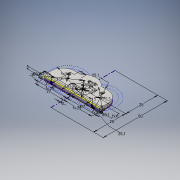
# Autodesk Inventor part: mount2
Saved by Autodesk Inventor 2016 (Build 200138000, 138)
## iProperties
Created: 2016-12-01
Part Number: mount2
Material: 一般
Document SubType Name: Modeling
Designer: KOTA-NPC2
Density: 1 g/cm^3
Appearance: 既定
Author: KOTA-NPC2
Autodesk Inventor part; units mm, degrees
ref_plane "YZ Plane" through (0, 0, 0) normal (1, 0, 0) x (0, 1, 0)
ref_plane "XZ Plane" through (0, 0, 0) normal (0, 1, 0) x (-1, 0, 0)
ref_plane "XY Plane" through (0, 0, 0) normal (0, 0, 1) x (1, 0, 0)
sketch "構築線" plane through (0, 0, 0) normal (0, 0, 1) x (1, 0, 0)
  circle A0 centre (0, 0) radius 8.5
  circle A1 centre (0, 0) radius 2.8 construction
  circle A2 centre (0, 0) radius 5 construction
  line L0 (0, -8.6) -> (-25, -8.6) construction
  line L1 (0, -11.6) -> (-25, -11.6) construction
  circle A3 centre (-12.8148, 0.95) radius 10.05 construction
  circle A4 centre (-12.8148, 0.95) radius 12.55 construction
  circle A5 centre (0, 5) radius 0.8
  circle A6 centre (-4.3301, 2.5) radius 0.8
  circle A7 centre (-4.3301, -2.5) radius 0.8
  circle A8 centre (0, -5) radius 0.8
  circle A9 centre (4.3301, -2.5) radius 0.8
  circle A10 centre (4.3301, 2.5) radius 0.8
  line L2 (25, -8.6) -> (0, -8.6) construction
  circle A11 centre (12.8148, 0.95) radius 10.05 construction
  circle A12 centre (12.8148, 0.95) radius 12.55 construction
  line L3 (0, -11.6) -> (25, -11.6) construction
  line L4 (-22, -8.6) -> (-22, -2.6)
  arc A13 (-13, 6.4) -> (-22, -2.6) centre (-13, -2.6) ccw
  line L5 (-13, 6.4) -> (-8, 6.4)
  line L6 (-22, -8.6) -> (0, -8.6)
  line L7 (0, 25) -> (0, -25)
  line L8 (0, -8.6) -> (22, -8.6)
  line L9 (22, -8.6) -> (22, -2.6)
  arc A14 (8, 6.4) -> (-8, 6.4) centre (0, 0) ccw
  line L10 (8, 6.4) -> (13, 6.4)
  arc A15 (22, -2.6) -> (13, 6.4) centre (13, -2.6) ccw
  circle A16 centre (0, 0) radius 3
  circle A17 centre (0, 0) radius 1
  circle A18 centre (12.8148, 0.95) radius 1.05
  circle A19 centre (-12.8148, 0.95) radius 1.05
  circle A20 centre (12.8148, 0.95) radius 2.75
  circle A21 centre (-12.8148, 0.95) radius 2.75
  dimension "d0" = 17
  dimension "d1" = 5.6
  dimension "d2" = 10
  dimension "d12" = 25
  dimension "d13" = 8.6
  dimension "d14" = 0
  dimension "d17" = 0
  dimension "d18" = 25
  dimension "d19" = 3
  dimension "d22" = 20.1
  dimension "d23" = 25.1
  dimension "d29" = 1.6
  dimension "d30" = 0
  dimension "d31" = 5
  dimension "d34" = 360
  dimension "d38" = 25
  dimension "d41" = 20.1
  dimension "d42" = 25.1
  dimension "d43" = 25
  dimension "d46" = 22
  dimension "d47" = 6
  dimension "d48" = 5
  dimension "d49" = 50
  dimension "d50" = 25
  dimension "d51" = 25
  dimension "d52" = 22
  dimension "d53" = 6
  dimension "d56" = 15
  dimension "d57" = 15
  dimension "d58" = 6
  dimension "d59" = 2
  dimension "d99" = 2.1
  dimension "d100" = 2.1
  dimension "d105" = 5.5
  dimension "d106" = 5.5
  constraints: 22 centre point, 22 end point, 10 coincident, 8 tangent, 7 horizontal, 6 point on circle, 2 concentric, 2 vertical, 1 collinear, 1 perpendicular, 1 point on line, 13 other
  measures "d0" diameter of A0
  measures "d1" diameter of A1
  measures "d2" diameter of A2
  measures "d12" distance of L0.start L0.end
  measures "d13" distance from line of point (0, 0) L0
  measures "d14" horizontal distance of point (0, 0) L0.start
  measures "d17" horizontal distance of L1.start point (0, 0)
  measures "d18" distance of L1.start L1.end
  measures "d19" distance between parallel lines of L1 L0
  measures "d22" diameter of A3
  measures "d23" diameter of A4
  measures "d29" diameter of A5
  measures "d30" horizontal distance of point (0, 0) A5.centre
  measures "d31" distance of point (0, 0) A5.centre
  measures "d38" distance of L0.start L2.start
  measures "d41" diameter of A11
  measures "d42" diameter of A12
  measures "d43" distance of L1.start L3.end
  measures "d46" distance of L0.start L4.start
  measures "d47" distance of L4.start L4.end
  measures "d48" distance of L5.start L5.end
  measures "d49" distance of L7.start L7.end
  measures "d50" distance of point (0, 0) L7.start
  measures "d51" distance of L7.end point (0, 0)
  measures "d52" distance of L0.start L8.end
  measures "d53" distance of L8.end L9.end
  measures "d56" distance between parallel lines of L8 L10
  measures "d57" distance between parallel lines of L6 L5
  measures "d58" diameter of A16
  measures "d59" diameter of A17
  measures "d99" diameter of A18
  measures "d100" diameter of A19
  measures "d105" diameter of A20
  measures "d106" diameter of A21
extrude "外形作成" add sketch "構築線" along normal blind 2.5 and the other way blind 1 contours A0 L7 A8 A16 A5 | A0 L7 A14 L10 A15 L9 L8 | L7 A5 A16 A8 A0 | A0 L7 L6 L4 A13 L5 A14 | A16 L7 A17 | L7 A17 A16 | A18 | A19 | A20 | A21
extrude "押し出し4" cut sketch "構築線" against normal blind 1 contours A0 L7 A8 A16 A5 | L7 A5 A16 A8 A0 | A16 L7 A17 | L7 A17 A16
sketch "固定具" plane through (-22, -8.6, 2.5) normal (0, -1, 0) x (1, 0, 0)
  circle A0 centre (6, -2) radius 1.05
  line L0 (0, 0) -> (0, -3.5) projected
  line L1 (0, 0) -> (44, 0) projected
  circle A1 centre (38, -2) radius 1.05
  point P0 (22, -2.5)
  dimension "d66" = 2.1
  dimension "d67" = 6
  dimension "d68" = 2
  dimension "d69" = 2.1
  dimension "d70" = 32
  dimension "d71" = 2
  constraints: 2 centre point
  measures "d66" diameter of A0
  measures "d67" distance from line of L0 A0.centre
  measures "d68" distance from line of L1 A0.centre
  measures "d69" diameter of A1
  measures "d70" distance of A1.centre A0.centre
  measures "d71" distance from line of L1 A1.centre
hole "穴1" at (16, -8.6, 0.5) direction (0, 1, 0) diameter 1.6 depth 3.5 tip angle 118
hole "穴2" at (-16, -8.6, 0.5) direction (0, 1, 0) diameter 1.6 depth 3.5 tip angle 118
extrude "押し出し5" cut sketch "構築線" along normal blind 2.1 contours A16 L7 A17 | L7 A17 A16
sketch "スケッチ6" plane through (0, 0, 2.5) normal (0, 0, 1) x (1, 0, 0)
  circle A0 centre (0, 0) radius 1 projected
  circle A1 centre (4.3301, 2.5) radius 0.8 projected
  circle A2 centre (4.3301, -2.5) radius 0.8 projected
  circle A3 centre (0, -5) radius 0.8 projected
  circle A4 centre (-4.3301, -2.5) radius 0.8 projected
  circle A5 centre (-4.3301, 2.5) radius 0.8 projected
  circle A6 centre (0, 5) radius 0.8 projected
  line L0 (-22, -8.6) -> (22, -8.6) construction
  line L1 (22, -8.6) -> (22, -2.6) construction
  arc A7 (22, -2.6) -> (13, 6.4) centre (13, -2.6) ccw construction
  line L2 (13, 6.4) -> (8, 6.4) construction
  arc A8 (8, 6.4) -> (-8, 6.4) centre (0, 0) ccw construction
  line L3 (-8, 6.4) -> (-13, 6.4) construction
  arc A9 (-13, 6.4) -> (-22, -2.6) centre (-13, -2.6) ccw construction
  line L4 (-22, -2.6) -> (-22, -8.6) construction
  line L5 (-22, -7.6) -> (22, -7.6)
  line L6 (-22, -2.6) -> (-22, -8.6) projected
  line L7 (-22, -7.6) -> (-22, -8.6)
  line L8 (22, -8.6) -> (-22, -8.6) projected
  line L9 (22, -8.6) -> (22, -7.6)
  dimension "d95" = 44
  dimension "d96" = 1
  constraints: 6 end point, 1 collinear, 1 horizontal, 1 perpendicular, 1 point on line
  measures "d95" distance of L5.start L5.end
  measures "d96" distance between parallel lines of L0 L5
extrude "押し出し6" add sketch "スケッチ6" along normal blind 0.5 contours L5 L9 L8 L6
extrude "押し出し7" cut sketch "構築線" against normal blind 1 and the other way blind 3 contours A18 | A19
extrude "押し出し8" cut sketch "構築線" along normal blind 1 and the other way blind 1 contours A20
extrude "押し出し9" cut sketch "構築線" along normal blind 1 and the other way blind 1 contours A21
equation "\"d18\" = d12"
